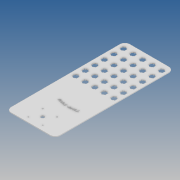
# Autodesk Inventor part: v1
Saved by Autodesk Inventor 2020 (Build 240168000, 168)
## iProperties
Created: 2021-04-16
Part Number: v1
Material: Generic
Document SubType Name: Modeling
Designer: stephen
Density: 1 g/cm^3
Appearance: Default
Author: stephen
Autodesk Inventor part; units mm, degrees
ref_plane "YZ Plane" through (0, 0, 0) normal (1, 0, 0) x (0, 1, 0)
ref_plane "XZ Plane" through (0, 0, 0) normal (0, 1, 0) x (-1, 0, 0)
ref_plane "XY Plane" through (0, 0, 0) normal (0, 0, 1) x (1, 0, 0)
sketch "Sketch1" plane through (0, 0, 0) normal (0, 1, 0) x (-1, 0, 0)
  line L0 (-64.77, -157.48) -> (64.77, -157.48)
  line L1 (64.77, -157.48) -> (64.77, 157.48)
  line L2 (64.77, 157.48) -> (-64.77, 157.48)
  line L3 (-64.77, 157.48) -> (-64.77, -157.48)
  line L4 (-64.77, -157.48) -> (64.77, 157.48) construction
  line L5 (64.77, -157.48) -> (-64.77, 157.48) construction
  point P0 (0, 0)
  dimension "d0" = 314.96
  dimension "d1" = 129.54
  constraints: 12 end point, 2 midpoint, 2 parallel, 1 horizontal, 1 perpendicular
  measures "d0" distance of L2.end L0.start
  measures "d1" distance of L1.end L2.end
extrude "Extrusion1" add sketch "Sketch1" along normal blind 1.5875
fillet "Fillet1" radius 12.7 4 edges at (64.77, 0.7937, 157.48) (-64.77, 0.7937, 157.48) (-64.77, 0.7937, -157.48) (64.77, 0.7937, -157.48)
sketch "Sketch2" plane through (0, 1.5875, 0) normal (0, 1, 0) x (1, 0, 0)
  line L0 (45.3645, 15.6325) -> (51.7145, 19.2987)
  line L1 (51.7145, 19.2987) -> (58.0645, 15.6325)
  line L2 (58.0645, 15.6325) -> (58.0645, 8.3002)
  line L3 (58.0645, 8.3002) -> (51.7145, 4.634)
  line L4 (51.7145, 4.634) -> (45.3645, 8.3002)
  line L5 (45.3645, 8.3002) -> (45.3645, 15.6325)
  line L6 (0, 0) -> (-19.5119, 0) construction
  line L7 (-19.5119, 0) -> (0, 0) construction
  line L8 (0, -19.1268) -> (0, 0) construction
  line L9 (19.9645, 15.6325) -> (26.3145, 19.2987)
  line L10 (19.9645, 8.3002) -> (19.9645, 15.6325)
  line L11 (26.3145, 4.634) -> (19.9645, 8.3002)
  line L12 (32.6645, 8.3002) -> (26.3145, 4.634)
  line L13 (32.6645, 15.6325) -> (32.6645, 8.3002)
  line L14 (26.3145, 19.2987) -> (32.6645, 15.6325)
  line L15 (-5.4355, 15.6325) -> (0.9145, 19.2987)
  line L16 (-5.4355, 8.3002) -> (-5.4355, 15.6325)
  line L17 (0.9145, 4.634) -> (-5.4355, 8.3002)
  line L18 (7.2645, 8.3002) -> (0.9145, 4.634)
  line L19 (7.2645, 15.6325) -> (7.2645, 8.3002)
  line L20 (0.9145, 19.2987) -> (7.2645, 15.6325)
  line L21 (-30.8355, 15.6325) -> (-24.4855, 19.2987)
  line L22 (-30.8355, 8.3002) -> (-30.8355, 15.6325)
  line L23 (-24.4855, 4.634) -> (-30.8355, 8.3002)
  line L24 (-18.1355, 8.3002) -> (-24.4855, 4.634)
  line L25 (-18.1355, 15.6325) -> (-18.1355, 8.3002)
  line L26 (-24.4855, 19.2987) -> (-18.1355, 15.6325)
  line L27 (-56.2355, 15.6325) -> (-49.8855, 19.2987)
  line L28 (-56.2355, 8.3002) -> (-56.2355, 15.6325)
  line L29 (-49.8855, 4.634) -> (-56.2355, 8.3002)
  line L30 (-43.5355, 8.3002) -> (-49.8855, 4.634)
  line L31 (-43.5355, 15.6325) -> (-43.5355, 8.3002)
  line L32 (-49.8855, 19.2987) -> (-43.5355, 15.6325)
  line L33 (45.3645, 41.0325) -> (51.7145, 44.6987)
  line L34 (45.3645, 33.7002) -> (45.3645, 41.0325)
  line L35 (51.7145, 30.034) -> (45.3645, 33.7002)
  line L36 (58.0645, 33.7002) -> (51.7145, 30.034)
  line L37 (58.0645, 41.0325) -> (58.0645, 33.7002)
  line L38 (51.7145, 44.6987) -> (58.0645, 41.0325)
  line L39 (19.9645, 41.0325) -> (26.3145, 44.6987)
  line L40 (19.9645, 33.7002) -> (19.9645, 41.0325)
  line L41 (26.3145, 30.034) -> (19.9645, 33.7002)
  line L42 (32.6645, 33.7002) -> (26.3145, 30.034)
  line L43 (32.6645, 41.0325) -> (32.6645, 33.7002)
  line L44 (26.3145, 44.6987) -> (32.6645, 41.0325)
  line L45 (-5.4355, 41.0325) -> (0.9145, 44.6987)
  line L46 (-5.4355, 33.7002) -> (-5.4355, 41.0325)
  line L47 (0.9145, 30.034) -> (-5.4355, 33.7002)
  line L48 (7.2645, 33.7002) -> (0.9145, 30.034)
  line L49 (7.2645, 41.0325) -> (7.2645, 33.7002)
  line L50 (0.9145, 44.6987) -> (7.2645, 41.0325)
  line L51 (-30.8355, 41.0325) -> (-24.4855, 44.6987)
  line L52 (-30.8355, 33.7002) -> (-30.8355, 41.0325)
  line L53 (-24.4855, 30.034) -> (-30.8355, 33.7002)
  line L54 (-18.1355, 33.7002) -> (-24.4855, 30.034)
  line L55 (-18.1355, 41.0325) -> (-18.1355, 33.7002)
  line L56 (-24.4855, 44.6987) -> (-18.1355, 41.0325)
  line L57 (-56.2355, 41.0325) -> (-49.8855, 44.6987)
  line L58 (-56.2355, 33.7002) -> (-56.2355, 41.0325)
  line L59 (-49.8855, 30.034) -> (-56.2355, 33.7002)
  line L60 (-43.5355, 33.7002) -> (-49.8855, 30.034)
  line L61 (-43.5355, 41.0325) -> (-43.5355, 33.7002)
  line L62 (-49.8855, 44.6987) -> (-43.5355, 41.0325)
  line L63 (45.3645, 66.4325) -> (51.7145, 70.0987)
  line L64 (45.3645, 59.1002) -> (45.3645, 66.4325)
  line L65 (51.7145, 55.434) -> (45.3645, 59.1002)
  line L66 (58.0645, 59.1002) -> (51.7145, 55.434)
  line L67 (58.0645, 66.4325) -> (58.0645, 59.1002)
  line L68 (51.7145, 70.0987) -> (58.0645, 66.4325)
  line L69 (19.9645, 66.4325) -> (26.3145, 70.0987)
  line L70 (19.9645, 59.1002) -> (19.9645, 66.4325)
  line L71 (26.3145, 55.434) -> (19.9645, 59.1002)
  line L72 (32.6645, 59.1002) -> (26.3145, 55.434)
  line L73 (32.6645, 66.4325) -> (32.6645, 59.1002)
  line L74 (26.3145, 70.0987) -> (32.6645, 66.4325)
  line L75 (-5.4355, 66.4325) -> (0.9145, 70.0987)
  line L76 (-5.4355, 59.1002) -> (-5.4355, 66.4325)
  line L77 (0.9145, 55.434) -> (-5.4355, 59.1002)
  line L78 (7.2645, 59.1002) -> (0.9145, 55.434)
  line L79 (7.2645, 66.4325) -> (7.2645, 59.1002)
  line L80 (0.9145, 70.0987) -> (7.2645, 66.4325)
  line L81 (-30.8355, 66.4325) -> (-24.4855, 70.0987)
  line L82 (-30.8355, 59.1002) -> (-30.8355, 66.4325)
  line L83 (-24.4855, 55.434) -> (-30.8355, 59.1002)
  line L84 (-18.1355, 59.1002) -> (-24.4855, 55.434)
  line L85 (-18.1355, 66.4325) -> (-18.1355, 59.1002)
  line L86 (-24.4855, 70.0987) -> (-18.1355, 66.4325)
  line L87 (-56.2355, 66.4325) -> (-49.8855, 70.0987)
  line L88 (-56.2355, 59.1002) -> (-56.2355, 66.4325)
  line L89 (-49.8855, 55.434) -> (-56.2355, 59.1002)
  line L90 (-43.5355, 59.1002) -> (-49.8855, 55.434)
  line L91 (-43.5355, 66.4325) -> (-43.5355, 59.1002)
  line L92 (-49.8855, 70.0987) -> (-43.5355, 66.4325)
  line L93 (45.3645, 91.8325) -> (51.7145, 95.4987)
  line L94 (45.3645, 84.5002) -> (45.3645, 91.8325)
  line L95 (51.7145, 80.834) -> (45.3645, 84.5002)
  line L96 (58.0645, 84.5002) -> (51.7145, 80.834)
  line L97 (58.0645, 91.8325) -> (58.0645, 84.5002)
  line L98 (51.7145, 95.4987) -> (58.0645, 91.8325)
  line L99 (19.9645, 91.8325) -> (26.3145, 95.4987)
  line L100 (19.9645, 84.5002) -> (19.9645, 91.8325)
  line L101 (26.3145, 80.834) -> (19.9645, 84.5002)
  line L102 (32.6645, 84.5002) -> (26.3145, 80.834)
  line L103 (32.6645, 91.8325) -> (32.6645, 84.5002)
  line L104 (26.3145, 95.4987) -> (32.6645, 91.8325)
  line L105 (-5.4355, 91.8325) -> (0.9145, 95.4987)
  line L106 (-5.4355, 84.5002) -> (-5.4355, 91.8325)
  line L107 (0.9145, 80.834) -> (-5.4355, 84.5002)
  line L108 (7.2645, 84.5002) -> (0.9145, 80.834)
  line L109 (7.2645, 91.8325) -> (7.2645, 84.5002)
  line L110 (0.9145, 95.4987) -> (7.2645, 91.8325)
  line L111 (-30.8355, 91.8325) -> (-24.4855, 95.4987)
  line L112 (-30.8355, 84.5002) -> (-30.8355, 91.8325)
  line L113 (-24.4855, 80.834) -> (-30.8355, 84.5002)
  line L114 (-18.1355, 84.5002) -> (-24.4855, 80.834)
  line L115 (-18.1355, 91.8325) -> (-18.1355, 84.5002)
  line L116 (-24.4855, 95.4987) -> (-18.1355, 91.8325)
  line L117 (-56.2355, 91.8325) -> (-49.8855, 95.4987)
  line L118 (-56.2355, 84.5002) -> (-56.2355, 91.8325)
  line L119 (-49.8855, 80.834) -> (-56.2355, 84.5002)
  line L120 (-43.5355, 84.5002) -> (-49.8855, 80.834)
  line L121 (-43.5355, 91.8325) -> (-43.5355, 84.5002)
  line L122 (-49.8855, 95.4987) -> (-43.5355, 91.8325)
  line L123 (45.3645, 117.2325) -> (51.7145, 120.8987)
  line L124 (45.3645, 109.9002) -> (45.3645, 117.2325)
  line L125 (51.7145, 106.234) -> (45.3645, 109.9002)
  line L126 (58.0645, 109.9002) -> (51.7145, 106.234)
  line L127 (58.0645, 117.2325) -> (58.0645, 109.9002)
  line L128 (51.7145, 120.8987) -> (58.0645, 117.2325)
  line L129 (19.9645, 117.2325) -> (26.3145, 120.8987)
  line L130 (19.9645, 109.9002) -> (19.9645, 117.2325)
  line L131 (26.3145, 106.234) -> (19.9645, 109.9002)
  line L132 (32.6645, 109.9002) -> (26.3145, 106.234)
  line L133 (32.6645, 117.2325) -> (32.6645, 109.9002)
  line L134 (26.3145, 120.8987) -> (32.6645, 117.2325)
  line L135 (-5.4355, 117.2325) -> (0.9145, 120.8987)
  line L136 (-5.4355, 109.9002) -> (-5.4355, 117.2325)
  line L137 (0.9145, 106.234) -> (-5.4355, 109.9002)
  line L138 (7.2645, 109.9002) -> (0.9145, 106.234)
  line L139 (7.2645, 117.2325) -> (7.2645, 109.9002)
  line L140 (0.9145, 120.8987) -> (7.2645, 117.2325)
  line L141 (-30.8355, 117.2325) -> (-24.4855, 120.8987)
  line L142 (-30.8355, 109.9002) -> (-30.8355, 117.2325)
  line L143 (-24.4855, 106.234) -> (-30.8355, 109.9002)
  line L144 (-18.1355, 109.9002) -> (-24.4855, 106.234)
  line L145 (-18.1355, 117.2325) -> (-18.1355, 109.9002)
  line L146 (-24.4855, 120.8987) -> (-18.1355, 117.2325)
  line L147 (-56.2355, 117.2325) -> (-49.8855, 120.8987)
  line L148 (-56.2355, 109.9002) -> (-56.2355, 117.2325)
  line L149 (-49.8855, 106.234) -> (-56.2355, 109.9002)
  line L150 (-43.5355, 109.9002) -> (-49.8855, 106.234)
  line L151 (-43.5355, 117.2325) -> (-43.5355, 109.9002)
  line L152 (-49.8855, 120.8987) -> (-43.5355, 117.2325)
  line L153 (45.3645, 142.6325) -> (51.7145, 146.2987)
  line L154 (45.3645, 135.3002) -> (45.3645, 142.6325)
  line L155 (51.7145, 131.634) -> (45.3645, 135.3002)
  line L156 (58.0645, 135.3002) -> (51.7145, 131.634)
  line L157 (58.0645, 142.6325) -> (58.0645, 135.3002)
  line L158 (51.7145, 146.2987) -> (58.0645, 142.6325)
  line L159 (19.9645, 142.6325) -> (26.3145, 146.2987)
  line L160 (19.9645, 135.3002) -> (19.9645, 142.6325)
  line L161 (26.3145, 131.634) -> (19.9645, 135.3002)
  line L162 (32.6645, 135.3002) -> (26.3145, 131.634)
  line L163 (32.6645, 142.6325) -> (32.6645, 135.3002)
  line L164 (26.3145, 146.2987) -> (32.6645, 142.6325)
  line L165 (-5.4355, 142.6325) -> (0.9145, 146.2987)
  line L166 (-5.4355, 135.3002) -> (-5.4355, 142.6325)
  line L167 (0.9145, 131.634) -> (-5.4355, 135.3002)
  line L168 (7.2645, 135.3002) -> (0.9145, 131.634)
  line L169 (7.2645, 142.6325) -> (7.2645, 135.3002)
  line L170 (0.9145, 146.2987) -> (7.2645, 142.6325)
  line L171 (-30.8355, 142.6325) -> (-24.4855, 146.2987)
  line L172 (-30.8355, 135.3002) -> (-30.8355, 142.6325)
  line L173 (-24.4855, 131.634) -> (-30.8355, 135.3002)
  line L174 (-18.1355, 135.3002) -> (-24.4855, 131.634)
  line L175 (-18.1355, 142.6325) -> (-18.1355, 135.3002)
  line L176 (-24.4855, 146.2987) -> (-18.1355, 142.6325)
  line L177 (-56.2355, 142.6325) -> (-49.8855, 146.2987)
  line L178 (-56.2355, 135.3002) -> (-56.2355, 142.6325)
  line L179 (-49.8855, 131.634) -> (-56.2355, 135.3002)
  line L180 (-43.5355, 135.3002) -> (-49.8855, 131.634)
  line L181 (-43.5355, 142.6325) -> (-43.5355, 135.3002)
  line L182 (-49.8855, 146.2987) -> (-43.5355, 142.6325)
  point P0 (51.7145, 11.9663)
  dimension "d5" = 12.7
  dimension "d8" = 25.4
  dimension "d11" = 25.4
  constraints: 366 end point, 2 horizontal, 1 collinear, 1 parallel, 1 perpendicular, 1 vertical, 361 other
  measures "d5" distance between parallel lines of L2 L5
  measures "d8" distance of L0.start L9.start
  measures "d11" distance of L0.start L33.start
extrude "Extrusion2" cut sketch "Sketch2" against normal blind 1.5875
sketch "Sketch3" plane through (0, 1.5875, 0) normal (0, 1, 0) x (1, 0, 0)
  circle A0 centre (0, -125.73) radius 4.445
  line L0 (19.05, -144.78) -> (-19.05, -144.78) construction
  line L1 (-19.05, -144.78) -> (-19.05, -106.68) construction
  line L2 (-19.05, -106.68) -> (19.05, -106.68) construction
  line L3 (19.05, -106.68) -> (19.05, -144.78) construction
  line L4 (19.05, -144.78) -> (-19.05, -106.68) construction
  line L5 (-19.05, -144.78) -> (19.05, -106.68) construction
  circle A1 centre (-19.05, -106.68) radius 1.5875
  circle A2 centre (-19.05, -144.78) radius 1.5875
  circle A3 centre (19.05, -144.78) radius 1.5875
  circle A4 centre (19.05, -106.68) radius 1.5875
  line L6 (0, 0) -> (0, -156.1828) construction
  line L7 (-52.07, -157.48) -> (52.07, -157.48) construction
  point P0 (0, -125.73)
  dimension "d17" = 38.1
  dimension "d18" = 12.7
  dimension "d19" = 3.175
  dimension "d20" = 8.89
  constraints: 14 end point, 5 centre point, 4 coincident, 3 equal radius, 3 midpoint, 2 parallel, 2 perpendicular, 1 horizontal, 1 point on line, 1 vertical
  measures "d17" distance of L0.end L1.end
  measures "d18" distance from line of L7 L0.start
  measures "d19" diameter of A3
  measures "d20" diameter of A0
extrude "Extrusion3" cut sketch "Sketch3" against normal blind 1.5875
sketch "Sketch4" plane through (0, 1.5875, 0) normal (0, 1, 0) x (1, 0, 0)
  arc A0 (-13.898, -61.2787) -> (36.902, -61.2787) centre (11.502, 17.7889) ccw
  line L0 (36.902, -61.2787) -> (-13.898, -61.2787) construction
  line L1 (34.7524, -61.9463) -> (34.0461, -67.2608)
  line L2 (34.0461, -67.2608) -> (36.2176, -66.6616)
  line L3 (36.2176, -66.6616) -> (36.0502, -67.912)
  line L4 (36.0502, -67.912) -> (29.8643, -69.619)
  line L5 (29.8643, -69.619) -> (30.0317, -68.3685)
  line L6 (30.0317, -68.3685) -> (32.2032, -67.7693)
  line L7 (32.2032, -67.7693) -> (32.9095, -62.4549)
  line L8 (32.9095, -62.4549) -> (34.7524, -61.9463)
  spline S0 degree 2 poles (26.4932, -63.7647) (28.0057, -63.495) (29.3421, -64.4611) (29.0666, -65.6743) knots 0 0 0 1 2 2 2
  line L9 (29.0666, -65.6743) -> (28.1206, -69.7971)
  line L10 (28.1206, -69.7971) -> (26.2385, -70.1327)
  line L11 (26.2385, -70.1327) -> (27.1612, -66.1044)
  spline S1 degree 2 poles (27.1612, -66.1044) (27.3168, -65.4293) (26.8769, -64.8755) (26.2106, -64.9943) knots 0 0 0 1 2 2 2
  spline S2 degree 2 poles (26.2106, -64.9943) (25.5638, -65.1096) (24.8079, -65.8515) (24.6469, -66.5526) knots 0 0 0 1 2 2 2
  line L12 (24.6469, -66.5526) -> (23.7242, -70.5809)
  line L13 (23.7242, -70.5809) -> (21.8421, -70.9165)
  line L14 (21.8421, -70.9165) -> (22.7841, -66.7994)
  spline S3 degree 2 poles (22.7841, -66.7994) (23.0581, -65.6065) (24.9369, -64.0421) (26.4932, -63.7647) knots 0 0 0 1 2 2 2
  line L15 (13.3384, -65.307) -> (15.2365, -65.1876)
  line L16 (15.2365, -65.1876) -> (13.7745, -69.3285)
  line L17 (13.7745, -69.3285) -> (16.1054, -66.5683)
  line L18 (16.1054, -66.5683) -> (17.407, -66.4865)
  line L19 (17.407, -66.4865) -> (17.8469, -69.0723)
  line L20 (17.8469, -69.0723) -> (19.3089, -64.9314)
  line L21 (19.3089, -64.9314) -> (21.1085, -64.8182)
  line L22 (21.1085, -64.8182) -> (18.9077, -71.0647)
  line L23 (18.9077, -71.0647) -> (16.7039, -71.2033)
  line L24 (16.7039, -71.2033) -> (16.1058, -68.2265)
  line L25 (16.1058, -68.2265) -> (13.3365, -71.4151)
  line L26 (13.3365, -71.4151) -> (11.1376, -71.5534)
  line L27 (11.1376, -71.5534) -> (13.3384, -65.307)
  line L28 (6.6227, -67.2824) -> (10.0152, -67.3733)
  line L29 (10.0152, -67.3733) -> (9.5058, -68.4962)
  line L30 (9.5058, -68.4962) -> (6.1132, -68.4054)
  line L31 (6.1132, -68.4054) -> (6.6227, -67.2824)
  line L32 (4.7756, -64.9942) -> (2.2198, -69.707)
  line L33 (2.2198, -69.707) -> (4.4621, -69.9219)
  line L34 (4.4621, -69.9219) -> (3.8596, -71.0304)
  line L35 (3.8596, -71.0304) -> (-2.5282, -70.4181)
  line L36 (-2.5282, -70.4181) -> (-1.9257, -69.3096)
  line L37 (-1.9257, -69.3096) -> (0.3167, -69.5245)
  line L38 (0.3167, -69.5245) -> (2.8726, -64.8118)
  line L39 (2.8726, -64.8118) -> (4.7756, -64.9942)
  spline S4 degree 2 poles (-3.5888, -63.7463) (-2.0797, -64.034) (-1.1759, -65.4133) (-1.866, -66.4484) knots 0 0 0 1 2 2 2
  line L40 (-1.866, -66.4484) -> (-4.2206, -69.9624)
  line L41 (-4.2206, -69.9624) -> (-6.0986, -69.6044)
  line L42 (-6.0986, -69.6044) -> (-3.7995, -66.1704)
  spline S5 degree 2 poles (-3.7995, -66.1704) (-3.4133, -65.5953) (-3.6267, -64.9209) (-4.2915, -64.7942) knots 0 0 0 1 2 2 2
  spline S6 degree 2 poles (-4.2915, -64.7942) (-4.9369, -64.6711) (-5.9077, -65.0946) (-6.3083, -65.6921) knots 0 0 0 1 2 2 2
  line L43 (-6.3083, -65.6921) -> (-8.6074, -69.1261)
  line L44 (-8.6074, -69.1261) -> (-10.4854, -68.7681)
  line L45 (-10.4854, -68.7681) -> (-8.1366, -65.2581)
  spline S7 degree 2 poles (-8.1366, -65.2581) (-7.455, -64.2414) (-5.1417, -63.4503) (-3.5888, -63.7463) knots 0 0 0 1 2 2 2
  line L46 (-16.4282, -60.4939) -> (-14.6124, -61.0596)
  line L47 (-14.6124, -61.0596) -> (-17.4555, -64.4064)
  line L48 (-17.4555, -64.4064) -> (-14.2932, -62.6595)
  line L49 (-14.2932, -62.6595) -> (-13.0481, -63.0474)
  line L50 (-13.0481, -63.0474) -> (-13.5597, -65.6199)
  line L51 (-13.5597, -65.6199) -> (-10.7166, -62.2732)
  line L52 (-10.7166, -62.2732) -> (-8.995, -62.8094)
  line L53 (-8.995, -62.8094) -> (-13.2795, -67.8597)
  line L54 (-13.2795, -67.8597) -> (-15.3878, -67.2029)
  line L55 (-15.3878, -67.2029) -> (-14.8845, -64.2087)
  line L56 (-14.8845, -64.2087) -> (-18.6091, -66.1995)
  line L57 (-18.6091, -66.1995) -> (-20.7127, -65.5442)
  line L58 (-20.7127, -65.5442) -> (-16.4282, -60.4939)
  point P0 (0, 0)
  constraints: 2 end point, 2 point on circle, 1 centre point, 1 horizontal, 1 other
extrude "Extrusion4" cut sketch "Sketch4" against normal blind 1.5875
body "Solid1"
